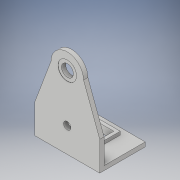
# Autodesk Inventor part: LampeSolaire2_LedAmoviblePart_Cover 3D printer
Saved by Autodesk Inventor 2019 (Build 230136000, 136)
## iProperties
Created: 2020-09-25
Part Number: LampeSolaire2_LedAmoviblePart_Cover 3D printer
Material: Generic
Document SubType Name: Modeling
Designer: nicolas
Density: 1 g/cm^3
Appearance: Default
Author: nicolas
## iProperties of the stored document LampeSolaire2_LedAmoviblePart_Cover_3DPrint.ipt
Created: 2020-10-22
Part Number: LampeSolaire2_LedAmoviblePart_Cover_3DPrint
Material: Generic
Document SubType Name: Modeling
Designer: nicolas
Density: 1 g/cm^3
Appearance: Default
Author: nicolas
Autodesk Inventor part; units mm, degrees
ref_plane "YZ Plane" through (0, 0, 0) normal (1, 0, 0) x (0, 1, 0)
ref_plane "XZ Plane" through (0, 0, 0) normal (0, 1, 0) x (-1, 0, 0)
ref_plane "XY Plane" through (0, 0, 0) normal (0, 0, 1) x (1, 0, 0)
sketch "Sketch2" plane through (-15, -30, 0) normal (0, 0, 1) x (1, 0, 0)
  arc A0 (22.5, 30) -> (7.5, 30) centre (15, 30) ccw
  line L0 (7.5, 30) -> (0, 10)
  line L1 (30, 10) -> (22.5, 30)
  line L2 (30, 0) -> (30, 10)
  line L3 (0, 10) -> (0, 0)
  line L4 (0, 0) -> (30, 0)
  circle A1 centre (15, 30) radius 2.75
  circle A2 centre (15, 8) radius 1.7
  line L5 (15, 30) -> (15, 8) construction
  line L6 (7.5, 30) -> (15, 30) construction
  dimension "d15" = 30
  dimension "d16" = 10
  dimension "d17" = 15
  dimension "d18" = 5.5
  dimension "d19" = 30
  dimension "d20" = 8
  dimension "d21" = 15
  dimension "d22" = 3.4
  constraints: 14 end point, 3 centre point, 2 equal length, 2 horizontal, 2 point on circle, 2 vertical, 1 coincident, 1 concentric, 1 parallel
  measures "d15" distance of L3.end L2.start
  measures "d16" distance of L0.end L3.end
  measures "d17" diameter of A0
  measures "d18" diameter of A1
  measures "d19" distance from line of A0.centre L4
  measures "d20" distance from line of L4 L5.end
  measures "d21" distance from line of L2 L5.end
  measures "d22" diameter of A2
extrude "Extrusion1" add sketch "Sketch2" along normal blind 2
sketch "Sketch3" plane through (-15, -30, 0) normal (0, -1, 0) x (1, 0, 0)
  line L0 (0, 0) -> (30, 0) projected
  line L1 (30, 0) -> (30, 2) projected
  line L2 (0, 2) -> (30, 2) projected
  line L3 (0, 0) -> (0, 2) projected
  point P0 (15, 0)
extrude "Extrusion2" add sketch "Sketch3" along normal blind 3.5
sketch "Sketch4" plane through (-15, -30, 0) normal (0, 0, -1) x (-1, 0, 0)
  line L0 (-30, 10) -> (-30, -3.5) projected
  line L1 (0, 10) -> (0, -3.5) projected
  line L2 (-30, -3.5) -> (0, -3.5)
  line L3 (0, -3.5) -> (0, -1.5)
  line L4 (0, -1.5) -> (-30, -1.5)
  line L5 (-30, -1.5) -> (-30, -3.5)
  point P0 (-15, 30)
  dimension "d27" = 2
  constraints: 8 end point, 2 parallel, 1 horizontal, 1 perpendicular, 1 point on line
  measures "d27" distance of L3.end L2.end
extrude "Extrusion3" add sketch "Sketch4" along normal blind 19
sketch "Sketch5" plane through (-15, -33.5, 0) normal (0, -1, 0) x (1, 0, 0)
  line L0 (10, -4.5) -> (20, -4.5)
  line L1 (20, -4.5) -> (20, -14.5)
  line L2 (20, -14.5) -> (10, -14.5)
  line L3 (10, -14.5) -> (10, -4.5)
  line L4 (10, -4.5) -> (20, -14.5) construction
  line L5 (20, -4.5) -> (10, -14.5) construction
  line L6 (15, 0) -> (15, -9.5) construction
  line L7 (30, 0) -> (0, 0) projected
  line L8 (30, -19) -> (0, -19) projected
  dimension "d31" = 10
  dimension "d32" = 9.5
  dimension "d33" = 10
  constraints: 14 end point, 3 midpoint, 2 parallel, 2 perpendicular, 1 horizontal
  measures "d31" distance of L0.end L1.end
  measures "d32" distance from line of L7 L6.end
  measures "d33" distance of L1.end L2.end
extrude "Extrusion4" cut sketch "Sketch5" against normal up to next
sketch "Sketch6" plane through (-15, -31.5, 0) normal (0, 1, 0) x (1, 0, 0)
  line L0 (20, 4.5) -> (10, 4.5) projected
  line L1 (20, 14.5) -> (20, 4.5) projected
  line L2 (10, 4.5) -> (10, 14.5) projected
  line L3 (10, 14.5) -> (20, 14.5) projected
  line L4 (21.5, 3) -> (8.5, 3)
  line L5 (8.5, 3) -> (8.5, 16)
  line L6 (8.5, 16) -> (21.5, 16)
  line L7 (21.5, 16) -> (21.5, 3)
  point P0 (15, 0)
  dimension "d36" = 1.5
  constraints: 8 end point, 3 other
  measures "d36" distance between parallel lines of L1 L7
extrude "Extrusion5" add sketch "Sketch6" along normal blind 1.5
sketch "Sketch7" plane through (-15, -30, 2) normal (0, 0, 1) x (1, 0, 0)
  circle A0 centre (15, 30) radius 4.275
  dimension "d39" = 8.55
  constraints: 1 centre point, 1 coincident
  measures "d39" diameter of A0
extrude "Extrusion6" cut sketch "Sketch7" against normal blind 0.1
body "Solid2"
